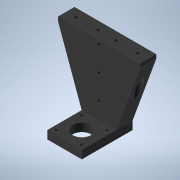
# Autodesk Inventor part: SliderMotorHalter
Saved by Autodesk Inventor 2021 (Build 250183000, 183)
## iProperties
Created: 2024-02-17
Part Number: SliderMotorHalter
Material: Generic
Document SubType Name: Modeling
Designer: Lukas
Density: 1 g/cm^3
Appearance: Default
Author: Lukas
Autodesk Inventor part; units mm, degrees
ref_plane "YZ Plane" through (0, 0, 0) normal (1, 0, 0) x (0, 1, 0)
ref_plane "XZ Plane" through (0, 0, 0) normal (0, 1, 0) x (-1, 0, 0)
ref_plane "XY Plane" through (0, 0, 0) normal (0, 0, 1) x (1, 0, 0)
sketch "Sketch1" plane through (0, 0, 0) normal (0, 0, 1) x (1, 0, 0)
  line L0 (-50, 45) -> (50, 45)
  line L1 (50, 45) -> (50, 40)
  line L2 (50, 40) -> (21, -40)
  line L3 (21, -40) -> (21, -50)
  line L4 (21, -50) -> (-21, -50)
  line L5 (-21, -50) -> (-21, -40)
  line L6 (-21, -40) -> (-50, 40)
  line L7 (-50, 40) -> (-50, 45)
  point P0 (0, 0)
  point P1 (0, -50)
  point P2 (0, 45)
  point P3 (-35.5, 0)
  dimension "d0" = 42
  dimension "d1" = 10
  dimension "d2" = 5
  dimension "d3" = 95
  dimension "d4" = 100
  constraints: 16 end point, 3 midpoint, 3 perpendicular, 2 equal length, 2 parallel, 2 vertical alignment, 1 horizontal, 1 horizontal alignment
  measures "d0" distance of L3.end L4.end
  measures "d1" distance of L2.end L3.end
  measures "d2" distance of L6.end L0.start
  measures "d3" distance between parallel lines of L0 L4
  measures "d4" distance of L0.start L0.end
extrude "Extrusion1" add sketch "Sketch1" along normal blind 20
sketch "Sketch2" plane through (-21, -50, 0) normal (0, -1, 0) x (1, 0, 0)
  line L0 (0, 20) -> (42, 20) projected
  line L1 (0, 0) -> (0, 20) projected
  line L2 (0, 20) -> (42, 20)
  line L3 (42, 20) -> (42, 62)
  line L4 (42, 62) -> (0, 62)
  line L5 (0, 62) -> (0, 20)
  circle A0 centre (21, 41) radius 11.25
  circle A1 centre (5.5, 56.5) radius 1.75
  circle A2 centre (5.5, 25.5) radius 1.75
  circle A3 centre (36.5, 25.5) radius 1.75
  circle A4 centre (36.5, 56.5) radius 1.75
  point P0 (21, 0)
  point P1 (21, 62)
  point P2 (0, 41)
  dimension "d7" = 22.5
  dimension "d8" = 31
  dimension "d9" = 31
  dimension "d10" = 15.5
  dimension "d11" = 15.5
  dimension "d12" = 3.5
  constraints: 8 end point, 5 centre point, 3 equal radius, 3 horizontal alignment, 3 vertical alignment, 2 midpoint, 2 parallel, 2 perpendicular, 1 horizontal
  measures "d7" diameter of A0
  measures "d8" distance of A4.centre A1.centre
  measures "d9" distance of A3.centre A4.centre
  measures "d10" horizontal distance of A0.centre A1.centre
  measures "d11" horizontal distance of A0.centre A4.centre
  measures "d12" diameter of A1
extrude "Extrusion2" add sketch "Sketch2" against normal blind 10
sketch "Sketch3" plane through (-21, -50, 0) normal (0, -1, 0) x (1, 0, 0)
  line L0 (71, 0) -> (-29, 0) projected
  line L1 (-29, 0) -> (-29, 20) projected
  line L2 (71, 20) -> (-29, 20) projected
  line L3 (71, 0) -> (71, 20) projected
  circle A0 centre (-17, 10) radius 5
  circle A1 centre (-17, 10) radius 2.15
  circle A2 centre (59, 10) radius 5
  circle A3 centre (59, 10) radius 2.15
  circle A4 centre (10, 10) radius 5
  circle A5 centre (32, 10) radius 5
  circle A6 centre (32, 10) radius 2.15
  circle A7 centre (10, 10) radius 2.15
  line L4 (0, 0) -> (0, 62) projected
  line L5 (42, 0) -> (42, 62) projected
  point P0 (21, 0)
  point P1 (-29, 10)
  dimension "d15" = 12
  dimension "d16" = 4.3
  dimension "d17" = 10
  dimension "d18" = 12
  dimension "d19" = 10
  dimension "d20" = 10
  constraints: 8 centre point, 6 equal radius, 4 coincident, 4 horizontal alignment, 1 midpoint
  measures "d15" distance from line of L1 A0.centre
  measures "d16" diameter of A1
  measures "d17" diameter of A0
  measures "d18" distance from line of L3 A2.centre
  measures "d19" distance from line of L4 A4.centre
  measures "d20" distance from line of L5 A5.centre
extrude "Extrusion3" cut sketch "Sketch3" against normal blind 92 contours A0 | A1 | A2 | A3 | A4 | A5 | A6 | A7
extrude "Extrusion5" cut sketch "Sketch3" against normal through all contours A1 | A3 | A6 | A7
sketch "Sketch4" plane through (0, 0, 20) normal (0, 0, 1) x (1, 0, 0)
  circle A0 centre (0, 40) radius 2.1
  circle A1 centre (0, 10) radius 2.1
  circle A2 centre (0, -20) radius 2.1
  line L0 (50, 45) -> (-50, 45) projected
  point P0 (0, 0)
  dimension "d23" = 5
  dimension "d24" = 30
  dimension "d25" = 30
  dimension "d26" = 4.2
  constraints: 3 centre point, 3 vertical alignment, 2 equal radius
  measures "d23" distance from line of L0 A0.centre
  measures "d24" distance of A1.centre A0.centre
  measures "d25" distance of A2.centre A1.centre
  measures "d26" diameter of A0
extrude "Extrusion4" cut sketch "Sketch4" against normal blind 10
equation "\"d9\" = d8"
equation "\"d10\" = 0.5 * d8"
equation "\"d11\" = 0.5 * d9"
equation "\"d18\" = d15"
equation "\"d20\" = d19"
body "Solid1"
